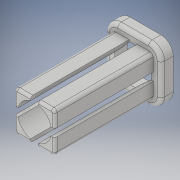
# Autodesk Inventor part: hjul-motor overgang nye motor
Saved by Autodesk Inventor 2019 (Build 230136000, 136)
## iProperties
Created: 2019-03-12
Part Number: hjul-motor overgang nye motor
Material: Generic
Document SubType Name: Modeling
Designer: jonas
Density: 1 g/cm^3
Appearance: Default
Author: jonas
Autodesk Inventor part; units mm, degrees
ref_plane "YZ Plane" through (0, 0, 0) normal (1, 0, 0) x (0, 1, 0)
ref_plane "XZ Plane" through (0, 0, 0) normal (0, 1, 0) x (-1, 0, 0)
ref_plane "XY Plane" through (0, 0, 0) normal (0, 0, 1) x (1, 0, 0)
sketch "Sketch1" plane through (0, 0, 0) normal (0, 0, 1) x (1, 0, 0)
  line L0 (-1.375, 1.625) -> (-0.3244, 1.625)
  line L1 (1.625, 1.375) -> (1.625, 0.3244)
  line L2 (1.375, -1.625) -> (0.3244, -1.625)
  line L3 (-1.625, -1.375) -> (-1.625, -0.3244)
  line L4 (0, -2.3475) -> (0, 2.3475) projected
  line L5 (-2.3475, 0) -> (2.3475, 0) projected
  arc A0 (-0.3244, 1.3413) -> (-1.3413, 0.3244) centre (0, 0) ccw
  line L6 (0.3244, 1.625) -> (0.3244, 1.3413)
  line L7 (0.3244, 1.625) -> (1.375, 1.625)
  line L8 (-0.3244, 1.3413) -> (-0.3244, 1.625)
  arc A1 (1.625, 1.375) -> (1.375, 1.625) centre (1.375, 1.375) ccw
  arc A2 (1.375, -1.625) -> (1.625, -1.375) centre (1.375, -1.375) ccw
  arc A3 (-1.625, -1.375) -> (-1.375, -1.625) centre (-1.375, -1.375) ccw
  arc A4 (-1.375, 1.625) -> (-1.625, 1.375) centre (-1.375, 1.375) ccw
  line L9 (-1.3413, -0.3244) -> (-1.625, -0.3244)
  line L10 (-1.625, 0.3244) -> (-1.3413, 0.3244)
  line L11 (0.3244, -1.3413) -> (0.3244, -1.625)
  line L12 (-0.3244, -1.625) -> (-0.3244, -1.3413)
  line L13 (1.3413, 0.3244) -> (1.625, 0.3244)
  line L14 (1.625, -0.3244) -> (1.3413, -0.3244)
  arc A5 (-1.3413, -0.3244) -> (-0.3244, -1.3413) centre (0, 0) ccw
  arc A6 (0.3244, -1.3413) -> (1.3413, -0.3244) centre (0, 0) ccw
  arc A7 (1.3413, 0.3244) -> (0.3244, 1.3413) centre (0, 0) ccw
  line L15 (1.625, -0.3244) -> (1.625, -1.375)
  line L16 (-0.3244, -1.625) -> (-1.375, -1.625)
  line L17 (-1.625, 0.3244) -> (-1.625, 1.375)
  dimension "d6" = 0.25
  dimension "d14" = 360
  dimension "d30" = 1.38
  dimension "d31" = 3.25
  constraints: 32 end point, 16 point on circle, 14 tangent, 9 parallel, 8 centre point, 4 perpendicular, 3 equal radius, 2 horizontal, 1 coincident, 27 other
  measures "d6" radius of A1
  measures "d30" radius of A7
  measures "d31" distance between parallel lines of L1 L17
extrude "Extrusion3" add sketch "Sketch1" along normal blind 8
sketch "Sketch2" plane through (0, 0, 0) normal (0, 0, -1) x (-1, 0, 0)
  line L0 (2.25, 2.25) -> (-2.25, 2.25)
  line L1 (-2.25, 2.25) -> (-2.25, -2.25)
  line L2 (-2.25, -2.25) -> (2.25, -2.25)
  line L3 (2.25, -2.25) -> (2.25, 2.25)
  line L4 (3.15, 0) -> (-3.15, 0) projected
  line L5 (0, -3.15) -> (0, 3.15) projected
  circle A0 centre (0, 0) radius 1.5
  dimension "d18" = 4.5
  dimension "d19" = 4.5
  dimension "d22" = 3
  constraints: 8 end point, 2 parallel, 1 centre point, 1 coincident, 1 horizontal, 1 perpendicular, 2 other
  measures "d18" distance between parallel lines of L1 L3
  measures "d19" distance between parallel lines of L2 L0
  measures "d22" diameter of A0
extrude "Extrusion5" add sketch "Sketch2" along normal blind 1 contours L3 L4 A0 L5 L0 | L5 A0 L4 L1 L0 | L3 L2 L5 A0 L4 | L4 A0 L5 L2 L1
fillet "Fillet1" radius 5 4 edges at (0.9758, 0.9758, 0) (-0.9758, 0.9758, 0) (-0.9758, -0.9758, 0) (0.9758, -0.9758, 0)
fillet "Fillet2" radius 1 4 edges at (-2.25, -2.25, -0.5) (-2.25, 2.25, -0.5) (2.25, -2.25, -0.5) (2.25, 2.25, -0.5)
fillet "Fillet3" radius 0.3 8 edges at (1.9571, 1.9571, 0) (2.25, 0, 0) (1.9571, -1.9571, 0) (0, -2.25, 0) (-1.9571, -1.9571, 0) (-2.25, 0, 0) (-1.9571, 1.9571, 0) (0, 2.25, 0)
fillet "Fillet4" radius 0.2 12 edges at (1.5518, -1.5518, 8) (0.8497, -1.625, 8) (1.625, -0.8497, 8) (0.8497, 1.625, 8) (1.625, 0.8497, 8) (1.5518, 1.5518, 8) (-1.5518, 1.5518, 8) (-1.625, 0.8497, 8) (-0.8497, 1.625, 8) (-1.5518, -1.5518, 8) (-0.8497, -1.625, 8) (-1.625, -0.8497, 8)
equation "\"d19\" = d18"
body "Solid3"
